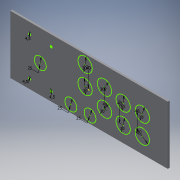
# Autodesk Inventor part: controles2
Saved by Autodesk Inventor 2016 (Build 200138000, 138)
## iProperties
Created: 2017-06-07
Part Number: controles2
Material: Generic
Document SubType Name: Modeling
Designer: fabio-note
Density: 1 g/cm^3
Appearance: Default
Author: fabio-note
Autodesk Inventor part; units mm, degrees
ref_plane "YZ Plane" through (0, 0, 0) normal (1, 0, 0) x (0, 1, 0)
ref_plane "XZ Plane" through (0, 0, 0) normal (0, 1, 0) x (-1, 0, 0)
ref_plane "XY Plane" through (0, 0, 0) normal (0, 0, 1) x (1, 0, 0)
sketch "Sketch1" plane through (0, 0, 0) normal (0, 1, 0) x (-1, 0, 0)
  line L0 (165, 61) -> (-165, 61)
  line L1 (-165, 61) -> (-165, -61)
  line L2 (-165, -61) -> (165, -61)
  line L3 (165, -61) -> (165, 61)
  point P0 (0, 0)
  point P1 (0, -61)
  point P2 (165, 0)
  dimension "d0" = 122
  dimension "d1" = 330
  constraints: 8 end point, 2 midpoint, 2 parallel, 1 horizontal, 1 horizontal alignment, 1 perpendicular, 1 vertical alignment
  measures "d0" distance between parallel lines of L2 L0
  measures "d1" distance between parallel lines of L1 L3
extrude "Extrusion1" add sketch "Sketch1" along normal blind 4
sketch "Esboço2" plane through (0, 0, 0) normal (0, -1, 0) x (1, 0, 0)
  circle A0 centre (111.4577, -28.224) radius 15
  circle A1 centre (71.1891, -28.224) radius 15
  circle A2 centre (71.1891, 11.776) radius 15
  circle A3 centre (111.4577, 11.776) radius 15
  circle A4 centre (31.9991, -18.8759) radius 15
  circle A5 centre (31.9991, 21.1241) radius 15
  circle A6 centre (-8.629, 1.9775) radius 15
  circle A7 centre (-8.629, 41.9775) radius 15
  circle A8 centre (1.7977, -45.4819) radius 12.5
  circle A9 centre (-38.4709, -45.4819) radius 12.5
  circle A10 centre (-102.5005, -2.2868) radius 12.5
  circle A11 centre (-79.7133, -42.1687) radius 2.25
  circle A12 centre (-124.8372, -42.1687) radius 2.25
  circle A13 centre (-79.7133, 38.8141) radius 2.1608
  circle A14 centre (-124.8372, 38.8141) radius 2.25
  point P0 (0, 0)
  dimension "d4" = 30
  dimension "d5" = 30
  dimension "d6" = 30
  dimension "d7" = 30
  dimension "d8" = 30
  dimension "d9" = 30
  dimension "d10" = 40
  dimension "d11" = 40
  dimension "d12" = 40
  dimension "d13" = 30
  dimension "d14" = 30
  dimension "d15" = 40
  dimension "d16" = 25
  dimension "d17" = 25
  dimension "d18" = 25
  dimension "d19" = 4.5
  dimension "d20" = 4.5
  dimension "d21" = 4.5
  constraints: 15 centre point
  measures "d4" diameter of A0
  measures "d5" diameter of A1
  measures "d6" diameter of A2
  measures "d7" diameter of A3
  measures "d8" diameter of A4
  measures "d9" diameter of A5
  measures "d10" distance of A2.centre A1.centre
  measures "d11" distance of A3.centre A0.centre
  measures "d12" distance of A5.centre A4.centre
  measures "d13" diameter of A6
  measures "d14" diameter of A7
  measures "d15" distance of A7.centre A6.centre
  measures "d16" diameter of A8
  measures "d17" diameter of A9
  measures "d18" diameter of A10
  measures "d19" diameter of A11
  measures "d20" diameter of A12
  measures "d21" diameter of A14
extrude "Extrusão2" cut sketch "Esboço2" against normal blind 5
sketch "Esboço3" plane through (0, 0, 0) normal (0, -1, 0) x (1, 0, 0)
  point P0 (0, 0)
body "Solid1"
